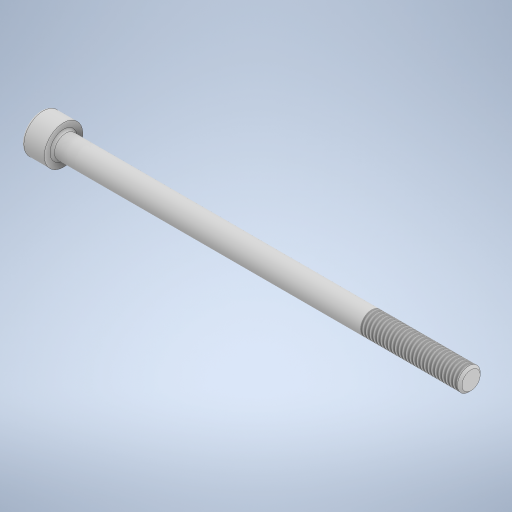
# Autodesk Inventor part: m5x90
Saved by Autodesk Inventor 2024 (Build 280153000, 153)
## iProperties
Created: 2025-12-15
Part Number: m5x90
Material: Generic
Document SubType Name: Modeling
Designer: schar
Density: 1 g/cm^3
Appearance: Default
Author: schar
Autodesk Inventor part; units mm, degrees
ref_plane "YZ Plane" through (0, 0, 0) normal (1, 0, 0) x (0, 1, 0)
ref_plane "XZ Plane" through (0, 0, 0) normal (0, 1, 0) x (-1, 0, 0)
ref_plane "XY Plane" through (0, 0, 0) normal (0, 0, 1) x (1, 0, 0)
sketch "Sketch1" plane through (0, 0, 0) normal (1, 0, 0) x (0, 1, 0)
  circle A0 centre (0, 0) radius 4.25
  dimension "d0" = 8.5
  constraints: 1 centre point, 1 coincident
  measures "d0" diameter of A0
extrude "Extrusion1" add sketch "Sketch1" along normal blind 5
sketch "Sketch2" plane through (5, 0, 0) normal (1, 0, 0) x (0, 0, -1)
  circle A0 centre (0, 0) radius 2.5
  dimension "d3" = 5
  constraints: 1 centre point, 1 coincident
  measures "d3" diameter of A0
extrude "Extrusion2" add sketch "Sketch2" along normal blind 90
thread "Thread1" size "M5x0.8" class "6g" standard "ANSI Metric M Profile" length 90 offset 68
chamfer "Chamfer1" distance 0.5 angle 45 1 edges at (95, 0, 2.5)
fillet "Fillet1" radius 0.5 1 edges at (5, 0, 2.5)
fillet "Fillet2" radius 0.5 1 edges at (0, -4.25, 0)
sketch "Sketch3" plane through (0, 0, 0) normal (-1, 0, 0) x (0, 0, 1)
  circle A0 centre (0, 0) radius 2
  line L0 (-1.1547, -2) -> (-2.3094, 0)
  line L1 (-2.3094, 0) -> (-1.1547, 2)
  line L2 (-1.1547, 2) -> (1.1547, 2)
  line L3 (1.1547, 2) -> (2.3094, 0)
  line L4 (2.3094, 0) -> (1.1547, -2)
  line L5 (1.1547, -2) -> (-1.1547, -2)
  point P0 (0, -2)
  dimension "d13" = 4
  constraints: 12 end point, 2 coincident, 1 midpoint, 1 vertical alignment, 15 other
extrude "Extrusion3" cut sketch "Sketch3" against normal blind 4
fillet "Fillet3" radius 0.5 6 edges at (4, 1, -1.7321) (4, 2, 0) (4, 1, 1.7321) (4, -1, 1.7321) (4, -2, 0) (4, -1, -1.7321)
body "Solid1"
